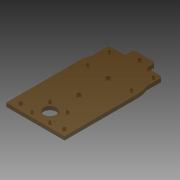
# Autodesk Inventor part: gearBoxBase
Saved by Autodesk Inventor 2013 (Build 170138000, 138)
## iProperties
Created: 2014-06-30
Part Number: gearBoxBase
Material: Polycarbonate, Smoke
Document SubType Name: Modeling
Designer: Nano
Density: 0.899 g/cm^3
Mass: 115.037 g
Surface Area: 451.851 cm^2
Volume: 127.961 cm^3
Author: Nano
Autodesk Inventor part; units mm, degrees
ref_plane "YZ Plane" through (0, 0, 0) normal (1, 0, 0) x (0, 1, 0)
ref_plane "XZ Plane" through (0, 0, 0) normal (0, 1, 0) x (-1, 0, 0)
ref_plane "XY Plane" through (0, 0, 0) normal (0, 0, 1) x (1, 0, 0)
sketch "Sketch1" plane through (0, 0, 0) normal (0, 1, 0) x (-1, 0, 0)
  line L0 (50.8, -50.8) -> (-50.8, -50.8)
  line L1 (-50.8, -50.8) -> (-50.8, 152.4)
  line L2 (-50.8, 152.4) -> (50.8, 152.4)
  line L3 (50.8, 152.4) -> (50.8, -50.8)
  point P0 (0, 0)
  dimension "d0" = 101.6
  dimension "d1" = 203.2
  constraints: 8 end point, 2 parallel, 1 horizontal, 1 perpendicular
  measures "d0" distance of L1.end L2.end
  measures "d1" distance of L0.end L1.end
extrude "Extrusion1" add sketch "Sketch1" along normal blind 6.35
sketch "Sketch2" plane through (0, 6.35, 0) normal (0, 1, 0) x (1, 0, 0)
  line L0 (-50.8, -152.4) -> (50.8, -152.4) projected
  line L1 (25.4, 0) -> (25.4, -152.4) construction
  circle A0 centre (0, -127) radius 11
  circle A1 centre (0, -76.2) radius 3.175
  circle A2 centre (0, -25.4) radius 3.175
  circle A3 centre (0, -127) radius 11 projected
  line L2 (50.8, -152.4) -> (50.8, 50.8) projected
  dimension "d4" = 22
  dimension "d5" = 6.35
  dimension "d6" = 50.8
  dimension "d7" = 25.4
  dimension "d10" = 6.35
  dimension "d11" = 50.8
  dimension "d12" = 22
  dimension "d13" = 50.8
  dimension "d14" = 50.8
  dimension "d15" = 50.8
  constraints: 3 centre point, 2 end point
  measures "d4" diameter of A0
  measures "d5" diameter of A1
  measures "d6" distance of A0.centre A1.centre
  measures "d7" distance from line of L0 A0.centre
  measures "d10" diameter of A2
  measures "d11" distance of A1.centre A2.centre
  measures "d12" diameter of A3
  measures "d13" distance from line of L2 A2.centre
  measures "d14" distance from line of L2 A1.centre
  measures "d15" distance from line of L2 A0.centre
extrude "Extrusion2" cut sketch "Sketch2" against normal through all
sketch "Sketch3" plane through (0, 6.35, 0) normal (0, 1, 0) x (1, 0, 0)
  circle A0 centre (15.5, -111.5) radius 2 projected
  circle A1 centre (15.5, -142.5) radius 2 projected
  circle A2 centre (-15.5, -142.5) radius 2 projected
  circle A3 centre (-15.5, -111.5) radius 2 projected
  point P0 (0, 0)
extrude "Extrusion3" cut sketch "Sketch3" against normal through all
sketch "Sketch4" plane through (0, 0, 0) normal (0, -1, 0) x (1, 0, 0)
  line L0 (50.8, 152.4) -> (-50.8, 152.4) projected
  line L1 (-50.8, 152.4) -> (-50.8, -50.8) projected
  circle A0 centre (-38.1, 139.7) radius 2.5146
  circle A1 centre (38.1, 139.7) radius 2.5146
  circle A2 centre (-38.1, -38.1) radius 2.5146
  circle A3 centre (38.1, -38.1) radius 2.5146
  point P0 (0, 0)
  dimension "d18" = 5.0292
  dimension "d19" = 12.7
  dimension "d20" = 12.7
  dimension "d23" = 76.2
  dimension "d26" = 177.8
  constraints: 4 centre point, 1 horizontal, 1 vertical, 6 other
  measures "d18" diameter of A0
  measures "d19" distance from line of L1 A0.centre
  measures "d20" distance from line of L0 A0.centre
  measures "d23" distance of A0.centre A1.centre
  measures "d26" distance of A0.centre A2.centre
extrude "Extrusion4" cut sketch "Sketch4" against normal through all
sketch "Sketch5" plane through (0, 6.35, 0) normal (0, 1, 0) x (1, 0, 0)
  circle A0 centre (-38.1, 15.24) radius 1.8542 projected
  circle A1 centre (-38.1, -22.86) radius 1.8542 projected
  circle A2 centre (38.1, 15.24) radius 1.8542 projected
  circle A3 centre (38.1, -22.86) radius 1.8542 projected
  point P0 (0, 0)
extrude "Extrusion5" cut sketch "Sketch5" against normal through all
sketch "Sketch7" plane through (0, 0, 0) normal (0, -1, 0) x (1, 0, 0)
  circle A0 centre (-38.1, -38.1) radius 2.5146 projected
  circle A1 centre (38.1, -38.1) radius 2.5146 projected
  circle A2 centre (0, 76.2) radius 3.175 projected
  circle A3 centre (0, 25.4) radius 3.175 projected
  line L0 (-50.8, -50.8) -> (50.8, -50.8) projected
  line L1 (50.8, -50.8) -> (50.8, 152.4) projected
  line L2 (-50.8, 152.4) -> (-50.8, -50.8) projected
  line L3 (-46.8468, -19.5288) -> (-46.8468, 5.7528)
  line L4 (46.8468, 5.7528) -> (46.8468, -19.5288)
  line L5 (16.1193, -38.1) -> (-16.1193, -38.1)
  line L6 (-19.2943, -34.925) -> (-19.2943, -22.7038)
  line L7 (19.2943, -22.7038) -> (19.2943, -34.925)
  line L8 (43.6718, -22.7038) -> (19.2943, -22.7038)
  line L9 (-19.2943, -22.7038) -> (-43.6718, -22.7038)
  line L10 (19.2943, -34.925) -> (16.1193, -38.1)
  line L11 (-19.2943, -34.925) -> (-16.1193, -38.1)
  line L12 (-43.6718, -22.7038) -> (-46.8468, -19.5288)
  line L13 (46.8468, -19.5288) -> (43.6718, -22.7038)
  arc A4 (-50.8, 25.4) -> (-46.8468, 5.7528) centre (0, 25.4) ccw
  arc A5 (46.8468, 5.7528) -> (50.8, 25.4) centre (0, 25.4) ccw
  arc A6 (3.1734, 76.1008) -> (-3.1734, 76.1008) centre (0, 25.4) ccw
  point P0 (0, 0)
  point P1 (46.8468, -22.7038)
  point P2 (-46.8468, -22.7038)
  point P3 (19.2943, -38.1)
  point P4 (-19.2943, -38.1)
  dimension "d41" = 19.2943
  dimension "d43" = 19.2943
  dimension "d44" = 3.175
  dimension "d45" = 3.175
  dimension "d46" = 3.175
  dimension "d47" = 3.175
  dimension "d48" = 3.175
  dimension "d49" = 3.175
  dimension "d50" = 3.175
  dimension "d51" = 3.175
  constraints: 22 end point, 10 point on line, 8 point on circle, 3 centre point, 3 horizontal, 3 perpendicular, 2 parallel, 2 tangent
  measures "d41" distance from line of A4.centre L7
  measures "d43" distance from line of A3.centre L6
  measures "d44" distance of L7.end point (19.294, -38.1)
  measures "d45" distance of L5.start point (19.294, -38.1)
  measures "d46" distance of L6.start point (-19.294, -38.1)
  measures "d47" distance of L5.end point (-19.294, -38.1)
  measures "d48" distance of L9.end point (-46.847, -22.704)
  measures "d49" distance of L3.start point (-46.847, -22.704)
  measures "d50" distance of L4.end point (46.847, -22.704)
  measures "d51" distance of L8.start point (46.847, -22.704)
extrude "Extrusion6" cut sketch "Sketch7" against normal through all contours L2 A4 L3 L12 L9 L6 L11 L5 L10 L7 L8 L13 L4 A5 L1 L0
sketch "Sketch8" plane through (0, 0, 0) normal (0, -1, 0) x (1, 0, 0)
  line L0 (-19.2943, -22.7038) -> (-19.2943, -34.925) projected
  line L1 (-16.1193, -38.1) -> (16.1193, -38.1) projected
  line L2 (19.2943, -34.925) -> (19.2943, -22.7038) projected
  circle A0 centre (0, -29.21) radius 2.5146
  point P0 (0, 0)
  dimension "d54" = 5.0292
  dimension "d55" = 8.89
  dimension "d56" = 19.2943
  dimension "d57" = 19.2943
  constraints: 1 centre point
  measures "d54" diameter of A0
  measures "d55" distance from line of L1 A0.centre
  measures "d56" distance from line of L2 A0.centre
  measures "d57" distance from line of L0 A0.centre
extrude "Extrusion7" cut sketch "Sketch8" against normal through all
equation "\"d4\" = d12"
equation "\"d14\" = d13"
equation "\"d15\" = d13"
equation "\"d43\" = d41"
equation "\"d45\" = d44"
equation "\"d46\" = d44"
equation "\"d47\" = d46"
equation "\"d48\" = d44"
equation "\"d49\" = d48"
equation "\"d50\" = d44"
equation "\"d51\" = d50"
equation "\"d56\" = d57"
body "Solid1"
